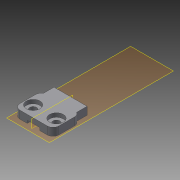
# Autodesk Inventor part: bed_belt_clip
Saved by Autodesk Inventor 2013 (Build 170138000, 138)
## iProperties
Created: 2014-01-31
Part Number: bed_belt_clip
Material: Ogólny
Document SubType Name: Modeling
Designer: Piotr
Density: 1 g/cm^3
Author: Piotr
Autodesk Inventor part; units mm, degrees
ref_plane "YZ Plane" through (0, 0, 0) normal (1, 0, 0) x (0, 1, 0)
ref_plane "XZ Plane" through (0, 0, 0) normal (0, 1, 0) x (-1, 0, 0)
ref_plane "XY Plane" through (0, 0, 0) normal (0, 0, 1) x (1, 0, 0)
ref_plane "Płaszczyzna konstrukcyjna1" through (0, 0, 0) normal (0, 0, 1) x (1, 0, 0)
sketch "Szkic1" plane through (0, 0, 0) normal (0, 0, 1) x (1, 0, 0)
  circle A0 centre (6, -50.25) radius 1.75 projected
  circle A1 centre (-6, -50.25) radius 1.75 projected
  circle A2 centre (6, -3.75) radius 1.75 construction
  circle A3 centre (-6, -3.75) radius 1.75 construction
  arc A4 (7, -56) -> (10, -53) centre (7, -53) ccw projected
  line L0 (10, -53) -> (10, -45) projected
  arc A5 (10, -45) -> (7, -42) centre (7, -45) ccw projected
  line L1 (7, -42) -> (5, -42) projected
  line L2 (5, -42) -> (5, -12) construction
  line L3 (5, -12) -> (7, -12) construction
  arc A6 (7, -12) -> (10, -9) centre (7, -9) ccw construction
  line L4 (10, -9) -> (10, -1) construction
  arc A7 (10, -1) -> (7, 2) centre (7, -1) ccw construction
  line L5 (7, 2) -> (-7, 2) construction
  arc A8 (-7, 2) -> (-10, -1) centre (-7, -1) ccw construction
  line L6 (-10, -1) -> (-10, -9) construction
  arc A9 (-10, -9) -> (-7, -12) centre (-7, -9) ccw construction
  line L7 (-7, -12) -> (-5, -12) construction
  line L8 (-5, -12) -> (-5, -42) construction
  line L9 (-5, -42) -> (-7, -42) projected
  arc A10 (-7, -42) -> (-10, -45) centre (-7, -45) ccw projected
  line L10 (-10, -45) -> (-10, -53) projected
  arc A11 (-10, -53) -> (-7, -56) centre (-7, -53) ccw projected
  line L11 (-7, -56) -> (7, -56) projected
  line L12 (-5.5, -42) -> (5.5, -42)
  line L13 (5.5, -42) -> (5.5, -37)
  line L14 (5.5, -37) -> (-5.5, -37)
  line L15 (-5.5, -37) -> (-5.5, -42)
  line L16 (0, -56) -> (0, 2) construction
  line L17 (-5.5, -37) -> (-8.5, -37)
  line L18 (-8.5, -37) -> (-8.5, -42)
  line L19 (-8.5, -42) -> (-5.5, -42)
  line L20 (-5.5, -42) -> (-5.5, -37)
  line L21 (5.5, -37) -> (8.5, -37)
  line L22 (8.5, -37) -> (8.5, -42)
  line L23 (8.5, -42) -> (5.5, -42)
  line L24 (5.5, -42) -> (5.5, -37)
  line L25 (-8.5, -42) -> (-8.5, -42.4019)
  line L26 (8.5, -42) -> (8.5, -42.4019)
  dimension "d0" = 11
  dimension "d1" = 3
  dimension "d2" = 3
  dimension "d3" = 5
  constraints: 30 end point, 8 parallel, 3 horizontal, 3 perpendicular, 2 collinear, 2 midpoint, 2 point on circle, 1 point on line, 1 other
  measures "d0" distance of L14.end L13.end
  measures "d1" distance of L19.end L18.end
  measures "d2" distance of L22.end L23.end
  measures "d3" distance of L21.end L22.end
extrude "Wyciągnięcie proste1" add sketch "Szkic1" along normal blind 4
ref_plane "Płaszczyzna konstrukcyjna2" through (0, -53, 0) normal (1, 0, 0) x (0, 0, -1)
sketch "Szkic2" plane through (0, -53, 0) normal (1, 0, 0) x (0, 0, -1)
  line L0 (0, -3) -> (-4, -3) projected
  line L1 (-4, -3) -> (-4, 16) projected
  line L2 (-4, 16) -> (0, 16) projected
  line L3 (0, 16) -> (0, -3) projected
  line L4 (-1.4, -3) -> (-1.4, -1) construction
  line L5 (-1.4, -3) -> (-1.4, -2.4)
  line L6 (-1.4, -2.4) -> (-1.2, -2.4)
  arc A0 (-1.2, -2.4) -> (-1.2, -1.6) centre (-1.2, -2) ccw
  line L7 (-1.2, -1.6) -> (-1.4, -1.6)
  line L8 (-1.4, -1.6) -> (-1.4, -1)
  line L9 (-1.4, -2) -> (-1.2, -2) construction
  line L10 (-1.4, -1) -> (0, -1)
  line L11 (0, -1) -> (0, -3)
  line L12 (0, -3) -> (-1.4, -3)
  point P0 (0, 53)
  dimension "d6" = 2
  dimension "d7" = 1.4
  dimension "d8" = 0.4
  dimension "d9" = 0.2
  constraints: 18 end point, 4 perpendicular, 4 point on line, 3 collinear, 2 point on circle, 2 tangent, 1 centre point, 1 midpoint, 1 parallel
  measures "d6" distance of L4.start L4.end
  measures "d7" distance between parallel lines of L4 L3
  measures "d8" radius of A0
  measures "d9" distance of L7.start L7.end
extrude "Wyciągnięcie proste2" cut sketch "Szkic2" along normal mid plane 6.5 contours L0 L5 L6 A0 L7 L8 L10 L3
pattern_linear "Szyk prostokątny1" count 10 spacing 2 along (0, 1, 0) of "Wyciągnięcie proste2"
sketch "Szkic3" plane through (0, 0, 4) normal (0, 0, 1) x (1, 0, 0)
  circle A0 centre (-6, -50.25) radius 1.75 projected
  circle A1 centre (6, -50.25) radius 1.75 projected
  circle A2 centre (-6, -50.25) radius 3.5
  circle A3 centre (6, -50.25) radius 3.5
  point P0 (0, 0)
  dimension "d15" = 7
  dimension "d16" = 7
  constraints: 2 centre point, 2 coincident
  measures "d15" diameter of A2
  measures "d16" diameter of A3
extrude "Wyciągnięcie proste3" cut sketch "Szkic3" against normal blind 2
sketch "Szkic4" plane through (0, 0, 0) normal (0, 0, -1) x (-1, 0, 0)
  line L0 (8.5, -37) -> (8.5, -42.4019) projected
  line L1 (3.25, -37) -> (8.5, -37) projected
  line L2 (-5.5, -42) -> (-5.5, -37) projected
  line L3 (-8.5, -42) -> (-5.5, -42) projected
  line L4 (5.5, -42) -> (5.5, -37) projected
  line L5 (8.5, -42) -> (5.5, -42) projected
  line L6 (-3.25, -56) -> (-3.25, -37) projected
  line L7 (-8.5, -37) -> (-3.25, -37) projected
  line L8 (-8.5, -42.4019) -> (-8.5, -37) projected
  arc A0 (-8.5, -42.4019) -> (-10, -45) centre (-7, -45) ccw projected
  line L9 (-10, -53) -> (-10, -45) projected
  arc A1 (-10, -53) -> (-7, -56) centre (-7, -53) ccw projected
  line L10 (-3.25, -56) -> (-7, -56) projected
  circle A2 centre (-6, -50.25) radius 1.75 projected
  line L11 (-8.5, -42) -> (-8.5, -37)
  line L12 (-8.5, -37) -> (-5.5, -37)
  point P0 (0, 0)
  constraints: 4 end point, 2 collinear
extrude "Wyciągnięcie proste4" add sketch "Szkic4" along normal blind 3 contours L0 L5 L4 L1 | L3 L8 L7 L2
